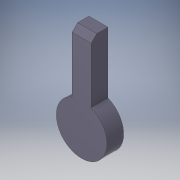
# Autodesk Inventor part: TARM10
Saved by Autodesk Inventor 2017 (Build 210142000, 142)
## iProperties
Created: 2018-11-17
Part Number: TARM10
Material: ABS Plastic
Document SubType Name: Modeling
Designer: Dell
Density: 1.06 g/cm^3
Appearance: Smooth - White
Author: Dell
Autodesk Inventor part; units mm, degrees
ref_plane "YZ Plane" through (0, 0, 0) normal (1, 0, 0) x (0, 1, 0)
ref_plane "XZ Plane" through (0, 0, 0) normal (0, 1, 0) x (-1, 0, 0)
ref_plane "XY Plane" through (0, 0, 0) normal (0, 0, 1) x (1, 0, 0)
sketch "Sketch3" plane through (0, 0, 0) normal (0, 0, 1) x (1, 0, 0)
  circle A0 centre (0, 0) radius 22.5
  line L0 (-8.5, 0) -> (8.5, 0)
  line L1 (8.5, 0) -> (8.5, 75.5)
  line L2 (8.5, 75.5) -> (-8.5, 75.5)
  line L3 (-8.5, 75.5) -> (-8.5, 0)
  dimension "d5" = 45
  dimension "d6" = 75.5
  dimension "d7" = 17
  constraints: 8 end point, 2 coincident, 2 parallel, 1 centre point, 1 horizontal, 1 midpoint, 1 perpendicular
  measures "d5" diameter of A0
  measures "d6" distance from line of point (0, 0) L2
  measures "d7" distance of L1.end L2.end
extrude "Extrusion3" add sketch "Sketch3" along normal blind 15
sketch "Sketch4" plane through (0, 0, 0) normal (0, 0, -1) x (-1, 0, 0)
  arc A0 (-8.5, 20.8327) -> (8.5, 20.8327) centre (0, 0) ccw projected
  line L0 (8.5, 75.5) -> (8.5, 20.8327) projected
  line L1 (-8.5, 75.5) -> (8.5, 75.5) projected
  line L2 (-8.5, 20.8327) -> (-8.5, 75.5) projected
  arc A1 (-6.5, 19.4422) -> (6.5, 19.4422) centre (0, 0) ccw
  line L3 (-6.5, 19.4422) -> (-6.5, 73.5)
  line L4 (-6.5, 73.5) -> (6.5, 73.5)
  line L5 (6.5, 73.5) -> (6.5, 19.4422)
  dimension "d10" = 2
  constraints: 6 end point, 2 point on circle, 1 centre point, 3 other
  measures "d10" radial gap between concentric circles of A0 A1
extrude "Extrusion4" cut sketch "Sketch4" against normal blind 13 contours L3 L4 L5 A1
chamfer "Chamfer1" distance 5 angle 45 1 edges at (0, 75.5, 15)
sketch "Sketch6" plane through (-8.5, 70.5, 15) normal (0, 0.7071068, 0.7071068) x (1, 0, 0)
  line L0 (2, 2.8284) -> (2, 4.2426) projected
  line L1 (2, 4.2426) -> (15, 4.2426) projected
  line L2 (15, 4.2426) -> (15, 2.8284) projected
  line L3 (15, 2.8284) -> (2, 2.8284) projected
  line L4 (0, 7.0711) -> (0, 0) projected
  line L5 (0, 0) -> (17, 0) projected
  line L6 (17, 0) -> (17, 7.0711) projected
  line L7 (17, 7.0711) -> (0, 7.0711) projected
  point P0 (8.5, -39.2444)
extrude "Extrusion5" add sketch "Sketch6" against normal blind 2 contours L0 L1 L2 L3 | L7 L6 L5 L4
body "Solid2"
